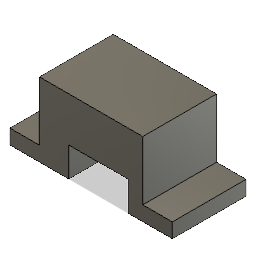
9589925d-ea7b-4d6d-85e0-95a7a58e631d (Autodesk Fusion 360 design; units mm, degrees)
Autodesk Fusion 360 part; units mm, degrees
sketch "Sketch1" plane through (0, 0, 0) normal (0, 0, 1) x (1, 0, 0)
  line L0 (110, 0) -> (80, 0)
  line L1 (80, 0) -> (80, 20)
  line L2 (80, 20) -> (40, 20)
  line L3 (40, 20) -> (40, 0)
  line L4 (0, 0) -> (40, 0)
  line L5 (80, 0) -> (110, 0)
  line L6 (110, 0) -> (110, 10)
  line L7 (110, 10) -> (90, 10)
  line L8 (90, 10) -> (90, 50)
  line L9 (90, 50) -> (20, 50)
  line L10 (0, 0) -> (0, 10)
  line L11 (0, 10) -> (20, 10)
  line L12 (20, 10) -> (20, 50)
  dimension "d1" = 110
  dimension "d2" = 30
  dimension "d3" = 20
  dimension "d4" = 40
  dimension "d5" = 10
  dimension "d6" = 20
  dimension "d7" = 70
  dimension "d8" = 10
  dimension "d9" = 20
  measures "d5" distance of L4.start
  measures "d8" distance of L4.start
extrude "Extrude1" add sketch "Sketch1" along normal blind 50
sketch "Sketch2" plane through (0, 0, 50) normal (0, 0, 1) x (1, 0, 0)
  line L0 (0, 0) -> (40, 0)
  line L1 (40, 0) -> (40, 20)
  line L2 (40, 20) -> (80, 20)
  line L3 (80, 20) -> (80, 0)
  line L4 (80, 0) -> (110, 0)
  line L5 (110, 0) -> (110, 10)
  line L6 (110, 10) -> (90, 10)
  line L7 (90, 10) -> (90, 50)
  line L8 (90, 50) -> (20, 50)
  line L9 (20, 50) -> (20, 10)
  line L10 (20, 10) -> (0, 10)
  line L11 (0, 10) -> (0, 0)
  line L12 (20, 50) -> (40, 50)
  line L13 (40, 50) -> (40, 40)
  line L14 (40, 40) -> (70, 40)
  line L15 (70, 40) -> (70, 50)
  line L16 (70, 50) -> (90, 50)
  dimension "d12" = 10
extrude "Extrude2" [rolled back] along distance -51 taper angle 0
sketch "Sketch3" plane through (0, 50, 0) normal (0, 1, 0) x (-1, 0, 0)
  line L0 (-40, 50) -> (-40, 0)
  line L1 (-40, 0) -> (-20, 0)
  line L2 (-20, 0) -> (-20, 50)
  line L3 (-20, 50) -> (-40, 50)
  line L4 (-90, 0) -> (-90, 50)
  line L5 (-20, 40) -> (-90, 40)
  line L6 (-20, 10) -> (-90, 10)
  dimension "d15" = 10
  dimension "d16" = 10
  measures "d16" distance of origin
extrude "Extrude3" [rolled back] along distance -20 taper angle 0
